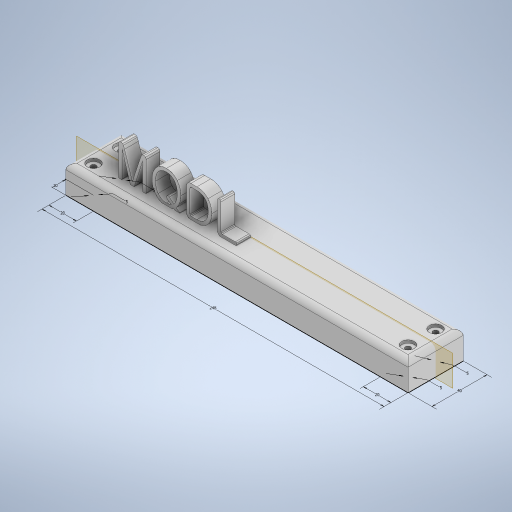
# Autodesk Inventor part: 윗대가리
Saved by Autodesk Inventor 2023 (Build 270158000, 158)
## iProperties
Created: 2023-08-31
Part Number: 윗대가리
Material: 일반
Document SubType Name: Modeling
Designer: rlatk
Density: 1 g/cm^3
Appearance: 기본값
Author: rlatk
Autodesk Inventor part; units mm, degrees
ref_plane "YZ Plane" through (0, 0, 0) normal (1, 0, 0) x (0, 1, 0)
ref_plane "XZ Plane" through (0, 0, 0) normal (0, 1, 0) x (-1, 0, 0)
ref_plane "XY Plane" through (0, 0, 0) normal (0, 0, 1) x (1, 0, 0)
sketch "스케치1" plane through (0, 0, 0) normal (0, 1, 0) x (-1, 0, 0)
  line L0 (124, -20) -> (-124, -20)
  line L1 (-124, -20) -> (-124, 20)
  line L2 (-124, 20) -> (124, 20)
  line L3 (124, 20) -> (124, -20)
  line L4 (124, -20) -> (-124, 20) construction
  line L5 (-124, -20) -> (124, 20) construction
  line L6 (124, -20) -> (104, -20)
  line L7 (104, -20) -> (104, 20)
  line L8 (104, 20) -> (124, 20)
  line L9 (124, 20) -> (124, -20)
  line L10 (-124, -20) -> (-104, -20)
  line L11 (-104, -20) -> (-104, 20)
  line L12 (-104, 20) -> (-124, 20)
  line L13 (-124, 20) -> (-124, -20)
  line L14 (0, -20) -> (0, 20)
  line L15 (124, 0) -> (-124, 0)
  circle A0 centre (114, 10) radius 2.5
  circle A1 centre (114, -10) radius 2.5
  circle A2 centre (-114, -10) radius 2.5
  circle A3 centre (-114, 10) radius 2.5
  point P0 (0, 0)
  dimension "d0" = 248
  dimension "d1" = 40
  dimension "d2" = 20
  dimension "d3" = 20
  dimension "d4" = 10
  dimension "d7" = 5
  dimension "d8" = 5
  dimension "d9" = 5
  dimension "d10" = 5
  constraints: 32 end point, 6 midpoint, 6 parallel, 4 centre point, 4 coincident, 3 horizontal, 3 perpendicular, 3 symmetric about line, 2 point on line
  measures "d0" distance of L1.end L2.end
  measures "d1" distance of L0.end L1.end
  measures "d2" distance of L7.end L8.end
  measures "d3" distance of L12.end L11.end
  measures "d4" distance from line of L2 point (114, 10)
  measures "d7" diameter of A0
  measures "d8" diameter of A1
  measures "d9" diameter of A2
  measures "d10" diameter of A3
extrude "돌출1" add sketch "스케치1" along normal blind 20 contours L0 L7 L15 L3 | L0 L14 L15 L7 | L15 L7 L2 L3 | L0 L11 L15 L14 | L15 L14 L2 L7 | L0 L1 L15 L11 | L15 L11 L2 L14 | L15 L1 L2 L11 | A0 | A1 | A2 | A3
extrude "돌출2" cut sketch "스케치1" along normal blind 10 contours A0 | A1 | A2 | A3
ref_plane "작업 평면1" through (-124, 0, 0) normal (0, 0, 1) x (1, 0, 0)
sketch "스케치3" plane through (-124, 0, 0) normal (0, 0, 1) x (1, 0, 0)
  point P0 (124, 0)
sketch "스케치4" plane through (-124, 0, 0) normal (0, 0, 1) x (1, 0, 0)
  line L0 (25.2416, 43.3184) -> (43.8453, 43.3184) construction
  line L1 (43.8453, 43.3184) -> (43.8453, 38.8306) construction
  line L2 (43.8453, 38.8306) -> (25.2416, 38.8306) construction
  line L3 (25.2416, 38.8306) -> (25.2416, 43.3184) construction
  line L4 (28.1489, 41.4936) -> (28.1489, 20.6019)
  spline S0 degree 2 poles (28.1489, 20.6019) (28.1489, 20.0143) (28.4736, 19.674) knots 0 0 0 1 1 1
  spline S1 degree 2 poles (28.4736, 19.674) (28.8911, 19.3184) (29.4014, 19.3184) knots 0 0 0 1 1 1
  spline S2 degree 2 poles (29.4014, 19.3184) (29.8963, 19.3184) (30.2519, 19.6431) knots 0 0 0 1 1 1
  spline S3 degree 2 poles (30.2519, 19.6431) (30.6695, 20.0143) (30.6695, 20.6019) knots 0 0 0 1 1 1
  line L5 (30.6695, 20.6019) -> (30.6695, 39.5452)
  line L6 (30.6695, 39.5452) -> (36.4994, 20.6328)
  spline S4 degree 2 poles (36.4994, 20.6328) (37.0715, 19.3184) (38.1385, 19.3184) knots 0 0 0 1 1 1
  spline S5 degree 2 poles (38.1385, 19.3184) (39.221, 19.3184) (39.7932, 20.6483) knots 0 0 0 1 1 1
  line L7 (39.7932, 20.6483) -> (45.6385, 39.5452)
  line L8 (45.6385, 39.5452) -> (45.6385, 20.6019)
  spline S6 degree 2 poles (45.6385, 20.6019) (45.6385, 20.0143) (45.9633, 19.674) knots 0 0 0 1 1 1
  spline S7 degree 2 poles (45.9633, 19.674) (46.3808, 19.3184) (46.8911, 19.3184) knots 0 0 0 1 1 1
  spline S8 degree 2 poles (46.8911, 19.3184) (47.4169, 19.3184) (47.7726, 19.6431) knots 0 0 0 1 1 1
  spline S9 degree 2 poles (47.7726, 19.6431) (48.1901, 20.0143) (48.1901, 20.6019) knots 0 0 0 1 1 1
  line L9 (48.1901, 20.6019) -> (48.1901, 41.4936)
  spline S10 degree 2 poles (48.1901, 41.4936) (48.1901, 42.2823) (47.7262, 42.6998) knots 0 0 0 1 1 1
  spline S11 degree 2 poles (47.7262, 42.6998) (47.2313, 43.2101) (46.5973, 43.2565) knots 0 0 0 1 1 1
  spline S12 degree 2 poles (46.5973, 43.2565) (45.9169, 43.3184) (45.3293, 42.9936) knots 0 0 0 1 1 1
  spline S13 degree 2 poles (45.3293, 42.9936) (44.7571, 42.5916) (44.5251, 41.772) knots 0 0 0 1 1 1
  line L10 (44.5251, 41.772) -> (43.9375, 40.1328)
  line L11 (43.9375, 40.1328) -> (38.1695, 22.7204)
  line L12 (38.1695, 22.7204) -> (32.4788, 40.071)
  line L13 (32.4788, 40.071) -> (31.7365, 42.205)
  spline S14 degree 2 poles (31.7365, 42.205) (31.5818, 42.6225) (31.1179, 42.9163) knots 0 0 0 1 1 1
  spline S15 degree 2 poles (31.1179, 42.9163) (30.453, 43.3184) (29.7416, 43.2874) knots 0 0 0 1 1 1
  spline S16 degree 2 poles (29.7416, 43.2874) (29.0767, 43.2101) (28.6282, 42.7771) knots 0 0 0 1 1 1
  spline S17 degree 2 poles (28.6282, 42.7771) (28.1489, 42.2978) (28.1489, 41.4936) knots 0 0 0 1 1 1
  line L14 (68.0767, 20.6792) -> (70.8602, 18.3751)
  spline S18 degree 2 poles (70.8602, 18.3751) (71.2932, 18.0658) (71.819, 18.0967) knots 0 0 0 1 1 1
  spline S19 degree 2 poles (71.819, 18.0967) (72.2829, 18.1895) (72.6231, 18.5606) knots 0 0 0 1 1 1
  spline S20 degree 2 poles (72.6231, 18.5606) (72.9014, 18.9163) (72.9014, 19.3338) knots 0 0 0 1 1 1
  spline S21 degree 2 poles (72.9014, 19.3338) (72.855, 19.8905) (72.453, 20.2153) knots 0 0 0 1 1 1
  line L15 (72.453, 20.2153) -> (69.9324, 22.1483)
  spline S22 degree 2 poles (69.9324, 22.1483) (71.4788, 23.5091) (72.3911, 25.9369) knots 0 0 0 1 1 1
  spline S23 degree 2 poles (72.3911, 25.9369) (73.288, 28.3802) (73.288, 31.3029) knots 0 0 0 1 1 1
  spline S24 degree 2 poles (73.288, 31.3029) (73.288, 36.2823) (70.7056, 39.5916) knots 0 0 0 1 1 1
  spline S25 degree 2 poles (70.7056, 39.5916) (67.8447, 43.2874) (62.8654, 43.2874) knots 0 0 0 1 1 1
  spline S26 degree 2 poles (62.8654, 43.2874) (57.8396, 43.2874) (55.1489, 39.7153) knots 0 0 0 1 1 1
  spline S27 degree 2 poles (55.1489, 39.7153) (52.4427, 36.2823) (52.4427, 31.3029) knots 0 0 0 1 1 1
  spline S28 degree 2 poles (52.4427, 31.3029) (52.4427, 26.4008) (54.9014, 23.571) knots 0 0 0 1 1 1
  spline S29 degree 2 poles (54.9014, 23.571) (57.8396, 19.3184) (62.8654, 19.3184) knots 0 0 0 1 1 1
  spline S30 degree 2 poles (62.8654, 19.3184) (64.4736, 19.3184) (66.0664, 19.7668) knots 0 0 0 1 1 1
  spline S31 degree 2 poles (66.0664, 19.7668) (67.4117, 20.138) (68.0767, 20.6792) knots 0 0 0 1 1 1
  line L16 (68.2777, 23.571) -> (64.9839, 26.3854)
  spline S32 degree 2 poles (64.9839, 26.3854) (64.5355, 26.7256) (64.1179, 26.6637) knots 0 0 0 1 1 1
  spline S33 degree 2 poles (64.1179, 26.6637) (63.5612, 26.5864) (63.221, 26.2462) knots 0 0 0 1 1 1
  spline S34 degree 2 poles (63.221, 26.2462) (62.8963, 25.8287) (62.8963, 25.3648) knots 0 0 0 1 1 1
  spline S35 degree 2 poles (62.8963, 25.3648) (62.9427, 24.839) (63.4994, 24.3905) knots 0 0 0 1 1 1
  line L17 (63.4994, 24.3905) -> (66.3138, 22.1947)
  spline S36 degree 2 poles (66.3138, 22.1947) (65.9891, 22.1328) (65.2004, 21.9163) knots 0 0 0 1 1 1
  spline S37 degree 2 poles (65.2004, 21.9163) (63.9324, 21.607) (62.8654, 21.607) knots 0 0 0 1 1 1
  spline S38 degree 2 poles (62.8654, 21.607) (59.0148, 21.607) (56.8963, 24.5452) knots 0 0 0 1 1 1
  spline S39 degree 2 poles (56.8963, 24.5452) (54.9633, 27.174) (54.9633, 31.3029) knots 0 0 0 1 1 1
  spline S40 degree 2 poles (54.9633, 31.3029) (54.9633, 35.54) (56.8963, 38.1534) knots 0 0 0 1 1 1
  spline S41 degree 2 poles (56.8963, 38.1534) (59.0148, 40.9988) (62.8654, 40.9988) knots 0 0 0 1 1 1
  spline S42 degree 2 poles (62.8654, 40.9988) (66.6849, 40.9988) (68.8035, 38.1534) knots 0 0 0 1 1 1
  spline S43 degree 2 poles (68.8035, 38.1534) (70.7674, 35.4936) (70.7674, 31.3029) knots 0 0 0 1 1 1
  spline S44 degree 2 poles (70.7674, 31.3029) (70.7674, 28.7204) (69.9478, 26.4472) knots 0 0 0 1 1 1
  spline S45 degree 2 poles (69.9478, 26.4472) (69.2674, 24.6844) (68.2777, 23.571) knots 0 0 0 1 1 1
  spline S46 degree 2 poles (80.6179, 42.7617) (79.087, 42.7617) (78.2056, 41.7411) knots 0 0 0 1 1 1
  spline S47 degree 2 poles (78.2056, 41.7411) (77.4324, 40.8441) (77.4324, 39.5143) knots 0 0 0 1 1 1
  line L18 (77.4324, 39.5143) -> (77.4324, 23.0452)
  spline S48 degree 2 poles (77.4324, 23.0452) (77.4324, 21.7462) (78.2056, 20.8493) knots 0 0 0 1 1 1
  spline S49 degree 2 poles (78.2056, 20.8493) (79.087, 19.8287) (80.6179, 19.8287) knots 0 0 0 1 1 1
  line L19 (80.6179, 19.8287) -> (84.9633, 19.8287)
  spline S50 degree 2 poles (84.9633, 19.8287) (90.0973, 19.8287) (93.0045, 23.2771) knots 0 0 0 1 1 1
  spline S51 degree 2 poles (93.0045, 23.2771) (95.7262, 26.4318) (95.7262, 31.3029) knots 0 0 0 1 1 1
  spline S52 degree 2 poles (95.7262, 31.3029) (95.7262, 36.1586) (93.0045, 39.3132) knots 0 0 0 1 1 1
  spline S53 degree 2 poles (93.0045, 39.3132) (90.0818, 42.7617) (84.9633, 42.7617) knots 0 0 0 1 1 1
  line L20 (84.9633, 42.7617) -> (80.6179, 42.7617)
  spline S54 degree 2 poles (80.9581, 22.1483) (80.4478, 22.1483) (80.2159, 22.4112) knots 0 0 0 1 1 1
  spline S55 degree 2 poles (80.2159, 22.4112) (79.953, 22.7359) (79.953, 23.1689) knots 0 0 0 1 1 1
  line L21 (79.953, 23.1689) -> (79.953, 39.3905)
  spline S56 degree 2 poles (79.953, 39.3905) (79.953, 39.8545) (80.2159, 40.1637) knots 0 0 0 1 1 1
  spline S57 degree 2 poles (80.2159, 40.1637) (80.4478, 40.4421) (80.9581, 40.4421) knots 0 0 0 1 1 1
  line L22 (80.9581, 40.4421) -> (84.9633, 40.4421)
  spline S58 degree 2 poles (84.9633, 40.4421) (88.8757, 40.4421) (91.4581, 37.6586) knots 0 0 0 1 1 1
  spline S59 degree 2 poles (91.4581, 37.6586) (93.1746, 35.2617) (93.1746, 31.3029) knots 0 0 0 1 1 1
  spline S60 degree 2 poles (93.1746, 31.3029) (93.1746, 27.3441) (91.2726, 24.9627) knots 0 0 0 1 1 1
  spline S61 degree 2 poles (91.2726, 24.9627) (88.8757, 22.1483) (84.9633, 22.1483) knots 0 0 0 1 1 1
  line L23 (84.9633, 22.1483) -> (80.9581, 22.1483)
  line L24 (99.855, 41.973) -> (99.855, 23.0452)
  spline S62 degree 2 poles (99.855, 23.0452) (99.855, 21.7462) (100.6282, 20.8493) knots 0 0 0 1 1 1
  spline S63 degree 2 poles (100.6282, 20.8493) (101.5097, 19.8287) (103.0406, 19.8287) knots 0 0 0 1 1 1
  line L25 (103.0406, 19.8287) -> (112.721, 19.8287)
  spline S64 degree 2 poles (112.721, 19.8287) (113.3241, 19.8287) (113.6798, 20.1844) knots 0 0 0 1 1 1
  spline S65 degree 2 poles (113.6798, 20.1844) (114.02, 20.5246) (114.02, 20.9885) knots 0 0 0 1 1 1
  spline S66 degree 2 poles (114.02, 20.9885) (114.02, 21.4679) (113.7107, 21.7771) knots 0 0 0 1 1 1
  spline S67 degree 2 poles (113.7107, 21.7771) (113.2932, 22.1483) (112.721, 22.1483) knots 0 0 0 1 1 1
  line L26 (112.721, 22.1483) -> (103.3808, 22.1483)
  spline S68 degree 2 poles (103.3808, 22.1483) (102.8705, 22.1483) (102.6385, 22.4112) knots 0 0 0 1 1 1
  spline S69 degree 2 poles (102.6385, 22.4112) (102.3757, 22.7359) (102.3757, 23.1689) knots 0 0 0 1 1 1
  line L27 (102.3757, 23.1689) -> (102.3757, 41.973)
  spline S70 degree 2 poles (102.3757, 41.973) (102.3757, 42.5916) (101.9581, 42.9627) knots 0 0 0 1 1 1
  spline S71 degree 2 poles (101.9581, 42.9627) (101.587, 43.2874) (101.1076, 43.2874) knots 0 0 0 1 1 1
  spline S72 degree 2 poles (101.1076, 43.2874) (100.5973, 43.2874) (100.1952, 42.9318) knots 0 0 0 1 1 1
  spline S73 degree 2 poles (100.1952, 42.9318) (99.855, 42.5916) (99.855, 41.973) knots 0 0 0 1 1 1
  point P0 (124, 0)
  constraints: 2 other
extrude "돌출3" add sketch "스케치4" along normal blind 10
fillet "모깎기1" radius 4 4 edges at (0, 20, 20) (124, 20, 0) (0, 20, -20) (-124, 20, 0)
sketch "스케치5" plane through (0, 20, 0) normal (0, 1, 0) x (1, 0, 0)
  circle A0 centre (-114, 10) radius 2.5 projected
  circle A1 centre (-114, -10) radius 2.5 projected
  circle A2 centre (114, -10) radius 2.5 projected
  circle A3 centre (114, 10) radius 2.5 projected
  point P0 (0, 0)
hole "구멍1" at (-114, 20, -10) at (-114, 20, 10) at (114, 20, 10) at (114, 20, -10) direction (0, -1, 0) diameter 3.6881 depth 22 tip angle 118 counterbore diameter 9 counterbore depth 2 thread size "M4.5x0.75" class "6H" standard "ISO Metric profile"
